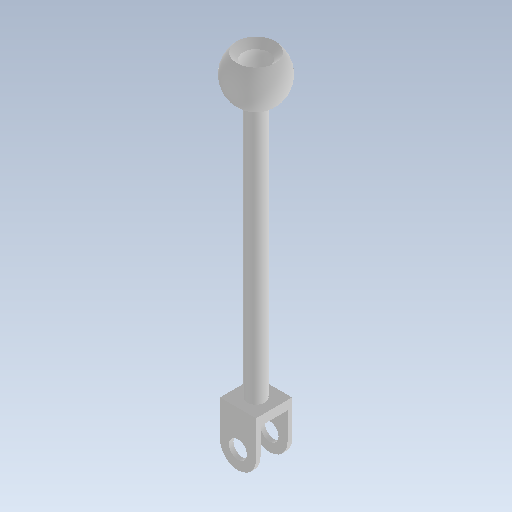
# Autodesk Inventor part: US_Dyad-01
Saved by Autodesk Inventor 2020.1 (Build 241239000, 239)
## iProperties
Created: 2019-10-24
Part Number: US_Dyad-01
Material: Generic
Document SubType Name: Modeling
Designer: sshel
Density: 1 g/cm^3
Appearance: Default
Author: sshel
Autodesk Inventor part; units mm, degrees
ref_plane "YZ Plane" through (0, 0, 0) normal (1, 0, 0) x (0, 1, 0)
ref_plane "XZ Plane" through (0, 0, 0) normal (0, 1, 0) x (-1, 0, 0)
ref_plane "XY Plane" through (0, 0, 0) normal (0, 0, 1) x (1, 0, 0)
sketch "Sketch1" plane through (0, 0, 0) normal (0, 1, 0) x (-1, 0, 0)
  line L0 (0, 0) -> (0, -776.116)
  line L1 (-50, -734.6946) -> (-50, 0)
  line L2 (0, 0) -> (-173.6931, 0)
  line L3 (0, 0) -> (0, 776.116)
  line L4 (-50, 734.6946) -> (-50, 0)
  arc A0 (-106.066, 982.182) -> (-50, 734.6946) centre (0, 876.116) ccw
  arc A1 (-70.7107, 946.8267) -> (0, 776.116) centre (0, 876.116) ccw
  line L5 (-70.7107, 946.8267) -> (-106.066, 982.182)
  line L6 (0, -1268.9888) -> (0, 1481.1208) construction
  line L7 (0, -776.116) -> (0, -876.116)
  line L8 (0, -876.116) -> (-50, -876.116)
  line L9 (-50, -876.116) -> (-50, -734.6946)
  point P0 (0, -2.2081)
  point P1 (-13.1062, 0)
  point P2 (-20, -18.7767)
  point P3 (-20, 3.1509)
  point P4 (-46.6023, 0)
  point P5 (-20, -18.7767)
  dimension "d6" = 45
  dimension "d7" = 50
  dimension "d8" = 100
  dimension "d9" = 50
  dimension "d10" = 1752.232
  constraints: 18 end point, 4 point on circle, 3 symmetric about line, 2 centre point, 2 horizontal, 2 point on line, 2 vertical, 1 coincident, 1 collinear, 1 perpendicular
  measures "d6" angle of L6 L5
  measures "d7" radial gap between concentric circles of A1 A0
  measures "d8" radius of A1
  measures "d9" distance between parallel lines of L4 L6
  measures "d10" distance of L7.end A1.centre
revolve "Revolution1" add sketch "Sketch1" angle 360 about axis through (0, 0, -10) along (0, 0, 1)
sketch "Sketch2" plane through (0, 0, 0) normal (0, 1, 0) x (-1, 0, 0)
  line L0 (50, -876.116) -> (-50, -876.116) projected
  arc A0 (-100, -876.116) -> (100, -876.116) centre (0, -876.116) ccw
  line L1 (65.0556, -876.116) -> (-85.3956, -876.116)
  line L2 (0, -338.7665) -> (0, -580.5318)
  line L3 (100, -876.116) -> (100, -676.116)
  line L4 (100, -676.116) -> (-100, -676.116)
  line L5 (-100, -676.116) -> (-100, -876.116)
  point P0 (0, 0)
  dimension "d11" = 100
  dimension "d12" = 200
  constraints: 10 end point, 4 point on line, 2 perpendicular, 2 point on circle, 2 vertical, 1 centre point, 1 horizontal, 1 midpoint, 1 tangent
  measures "d11" radius of A0
  measures "d12" distance of L5.end L4.end
extrude "Extrusion1" add sketch "Sketch2" along normal mid plane 200
sketch "Sketch4" plane through (0, 0, 0) normal (0, 1, 0) x (-1, 0, 0)
  arc A0 (-100, -876.116) -> (100, -876.116) centre (0, -876.116) ccw construction
  circle A1 centre (0, -876.116) radius 50
  point P0 (0, 0)
  dimension "d16" = 50
  constraints: 1 centre point, 1 coincident
  measures "d16" radius of A1
extrude "Extrusion2" cut sketch "Sketch4" along normal through all both and the other way through all
sketch "Sketch6" plane through (0, 0, 0) normal (1, 0, 0) x (0, 1, 0)
  line L0 (-100, -976.116) -> (100, -976.116) construction
  line L1 (0, -623.7458) -> (0, -465.1617)
  line L2 (75, -976.116) -> (-75, -976.116)
  line L3 (-75, -976.116) -> (-75, -726.116)
  line L4 (-75, -726.116) -> (75, -726.116)
  line L5 (75, -726.116) -> (75, -976.116)
  point P0 (0, 0)
  point P1 (0, -976.116)
  dimension "d27" = 150
  dimension "d28" = 250
  constraints: 10 end point, 2 parallel, 1 collinear, 1 horizontal, 1 midpoint, 1 perpendicular, 1 point on line, 1 vertical, 1 other
  measures "d27" distance between parallel lines of L3 L5
  measures "d28" distance of L2.end L3.end
extrude "Extrusion4" cut sketch "Sketch6" along normal through all both and the other way through all
equation "\"d7\" = rod_radius"
equation "\"d8\" = S_radius"
equation "\"d9\" = rod_radius"
equation "\"d10\" = L1"
equation "\"d11\" = S_radius"
equation "\"d12\" = 2 * S_radius"
equation "\"d13\" = 2 * S_radius"
equation "\"d16\" = rod_radius"
equation "\"d27\" = 3 * rod_radius"
equation "\"d28\" = 5 * rod_radius"
equation "\"L1\" = 1752.23201"
equation "\"rod_radius\" = 50"
equation "\"S_radius\" = 2 * rod_radius"
equation "\"dyad1_Fx\" = -4260.66351"
equation "\"dyad1_Fy\" = 914.69194"
equation "\"dyad1_Fz\" = 2675.35545"
equation "\"dyad2_Fx\" = -451.87793"
equation "\"dyad2_Fy\" = -915.49296"
equation "\"dyad2_Fz\" = 3417.84038"
equation "\"dyad3_Fx\" = -4318"
equation "\"dyad3_Fz\" = 1248"
equation "\"dyad4_Fx\" = 2692.78997"
equation "\"dyad4_Fy\" = 2100.31348"
equation "\"dyad4_Fz\" = 2764.89028"
equation "\"dyad5_Fx\" = -406.72783"
equation "\"dyad5_Fy\" = 1152.9052"
equation "\"dyad5_Fz\" = 2892.96636"
equation "\"L2\" = 1260.47471"
equation "\"L3\" = 1299.40028"
equation "\"L4\" = 3944.54642"
equation "\"L5\" = 4863.26059"
body "Solid1"
